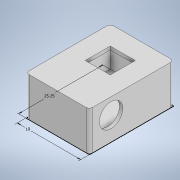
# Autodesk Inventor part: carcasaXeotype_BUTTON
Saved by Autodesk Inventor 2020 (Build 240168000, 168)
## iProperties
Created: 2021-04-10
Part Number: carcasaXeotype_BUTTON
Material: Generic
Document SubType Name: Modeling
Designer: Vlasciar
Density: 1 g/cm^3
Appearance: Default
Author: Vlasciar
Autodesk Inventor part; units mm, degrees
ref_plane "YZ Plane" through (0, 0, 0) normal (1, 0, 0) x (0, 1, 0)
ref_plane "XZ Plane" through (0, 0, 0) normal (0, 1, 0) x (-1, 0, 0)
ref_plane "XY Plane" through (0, 0, 0) normal (0, 0, 1) x (1, 0, 0)
sketch "Sketch1" plane through (0, 0, 0) normal (0, 1, 0) x (-1, 0, 0)
  line L0 (-9.5, -12.625) -> (9.5, -12.625)
  line L1 (9.5, -12.625) -> (9.5, 12.625)
  line L2 (9.5, 12.625) -> (-9.5, 12.625)
  line L3 (-9.5, 12.625) -> (-9.5, -12.625)
  line L4 (-9.5, -12.625) -> (9.5, 12.625) construction
  line L5 (9.5, -12.625) -> (-9.5, 12.625) construction
  point P0 (0, 0)
  dimension "d0" = 19
  dimension "d1" = 25.25
  constraints: 12 end point, 2 midpoint, 2 parallel, 1 horizontal, 1 perpendicular
  measures "d0" distance of L1.end L2.end
  measures "d1" distance of L0.end L1.end
extrude "Extrusion1" add sketch "Sketch1" along normal blind 10.75
shell "Shell1" thickness 1 removed faces 1 at (3.1667, 10.75, 4.2083)
sketch "Sketch2" plane through (9.5, 0, 12.625) normal (1, 0, 0) x (0, 0, -1)
  line L0 (1, 1) -> (24.25, 1) projected
  circle A0 centre (6.5, 7) radius 3.5
  line L1 (1, 1) -> (1, 10.75) projected
  line L2 (2, 3.75) -> (5.201, 3.75)
  line L3 (7.799, 3.75) -> (24, 3.75)
  point P0 (12.625, 0)
  dimension "d6" = 7
  dimension "d8" = 2
  constraints: 4 end point, 2 point on circle, 1 centre point, 1 coincident
  measures "d6" diameter of A0
  measures "d8" distance edge to line of A0 L1
extrude "Extrusion2" cut sketch "Sketch2" against normal blind 10.75
sketch "Sketch3" plane through (0, 10.75, 0) normal (0, 1, 0) x (1, 0, 0)
  line L0 (-8.5, -11.625) -> (-8.5, 11.625) projected
  line L1 (-8.5, 11.625) -> (8.5, 11.625) projected
  line L2 (-9.5, -12.625) -> (9.5, -12.625) projected
  line L3 (9.5, -12.625) -> (9.5, 12.625) projected
  line L4 (9.5, 12.625) -> (-9.5, 12.625) projected
  line L5 (-9.5, 12.625) -> (-9.5, -12.625) projected
  line L6 (-9.5, -12.625) -> (9.5, -12.625)
  line L7 (9.5, -12.625) -> (9.5, 12.625)
  line L8 (9.5, 12.625) -> (-9.5, 12.625)
  line L9 (-9.5, 12.625) -> (-9.5, -12.625)
  line L10 (3.75, 6.875) -> (-3.75, 6.875)
  line L11 (-3.75, 6.875) -> (-3.75, -0.625)
  line L12 (-3.75, -0.625) -> (3.75, -0.625)
  line L13 (3.75, -0.625) -> (3.75, 6.875)
  line L14 (3.75, 6.875) -> (-3.75, -0.625) construction
  line L15 (-3.75, 6.875) -> (3.75, -0.625) construction
  point P0 (0, 0)
  point P1 (0, 3.125)
  dimension "d11" = 8.5
  dimension "d12" = 8.5
  dimension "d13" = 7.5
  dimension "d14" = 7.5
  constraints: 20 end point, 4 parallel, 2 horizontal, 2 midpoint, 2 perpendicular
  measures "d11" distance from line of L0 point (0, 3.125)
  measures "d12" distance from line of L1 point (0, 3.125)
  measures "d13" distance of L12.end L11.end
  measures "d14" distance of L10.end L11.end
extrude "Extrusion3" add sketch "Sketch3" along normal blind 1
fillet "Fillet1" radius 1 4 edges at (9.5, 5.875, -12.625) (-9.5, 5.875, -12.625) (-9.5, 5.875, 12.625) (9.5, 5.875, 12.625)
body "Solid1"
